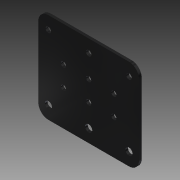
# Autodesk Inventor part: 30287-01
Saved by Autodesk Inventor 2014 (Build 180170000, 170)
## iProperties
Category: NS
Created: 2012-10-15
Part Number: 30287-01
Material: Steel, Mild
Document SubType Name: Modeling
Designer: Edward
Density: 7.86 g/cm^3
Mass: 87.1512 g
Surface Area: 222.023 cm^2
Volume: 32.1591 cm^3
Appearance: Lacquer - Black
Description: Spindle Mount Plate (12ga)
Project: Shapeoko
Vendor: ProkTech
User Status: F
Stock Number: S2SM-01
Authority: PER BARRY PROCK 8-22-13
Author: Edward
Subject: Structural
Comments: Fusion
Title: Spindle Mount Plate
Autodesk Inventor part; units mm, degrees
ref_plane "YZ Plane" through (0, 0, 0) normal (1, 0, 0) x (0, 1, 0)
ref_plane "XZ Plane" through (0, 0, 0) normal (0, 1, 0) x (-1, 0, 0)
ref_plane "XY Plane" through (0, 0, 0) normal (0, 0, 1) x (1, 0, 0)
sketch "Sketch1" plane through (0, 0, 0) normal (0, 0, 1) x (1, 0, 0)
  line L0 (-50, 45) -> (50, 45)
  line L1 (50, 45) -> (50, -45)
  line L2 (50, -45) -> (-50, -45)
  line L3 (-50, -45) -> (-50, 45)
  point P0 (0, 0)
  dimension "d0" = 100
  dimension "d1" = 90
  dimension "d2" = 50
  dimension "d3" = 45
  constraints: 8 end point, 2 parallel, 1 horizontal, 1 perpendicular
  measures "d0" distance of L1.end L2.end
  measures "d1" distance of L0.end L1.end
  measures "d2" distance from line of point (0, 0) L3
  measures "d3" distance from line of L0 point (0, 0)
extrude "Extrusion1" add sketch "Sketch1" along normal blind 2.6568
fillet "Fillet1" radius 10 4 edges at (50, 45, 1.3284) (-50, 45, 1.3284) (50, -45, 1.3284) (-50, -45, 1.3284)
sketch "Sketch2" plane through (0, 0, 2.6568) normal (0, 0, 1) x (1, 0, 0)
  line L0 (50, 35) -> (50, -35) projected
  line L1 (-40, 45) -> (40, 45) projected
  circle A0 centre (40, 32.3) radius 2.75
  circle A1 centre (40, -32.3) radius 3.5685
  point P0 (0, 0)
  dimension "d7" = 5.5
  dimension "d8" = 10
  dimension "d10" = 7.137
  dimension "d12" = 10
  dimension "d52" = 64.6
  dimension "d53" = 12.7
  constraints: 2 centre point
  measures "d7" diameter of A0
  measures "d8" distance from line of L0 A0.centre
  measures "d10" diameter of A1
  measures "d12" distance from line of L0 A1.centre
  measures "d52" distance of A1.centre A0.centre
  measures "d53" distance from line of L1 A0.centre
extrude "Extrusion2" cut sketch "Sketch2" against normal through all
pattern_linear "Rectangular Pattern1" count 3 spacing 40 along (-1, 0, 0) of "Extrusion2"
sketch "Sketch3" plane through (0, 0, 2.6568) normal (0, 0, 1) x (1, 0, 0)
  line L0 (40, -45) -> (-40, -45) projected
  line L1 (-50, -35) -> (-50, 35) projected
  circle A0 centre (-25, -10) radius 2.6
  point P0 (0, 0)
  dimension "d18" = 5.2
  dimension "d19" = 25
  dimension "d20" = 35
  constraints: 1 centre point
  measures "d18" diameter of A0
  measures "d19" distance from line of L1 A0.centre
  measures "d20" distance from line of L0 A0.centre
extrude "Extrusion3" cut sketch "Sketch3" against normal through all
pattern_linear "Rectangular Pattern2" count 3 spacing 25 along (1, 0, 0) count 2 spacing 20 along (0, 1, 0) of "Extrusion3"
equation "\"d2\" = 0.5 * d0"
equation "\"d3\" = 0.5 * d1"
body "Solid1"
